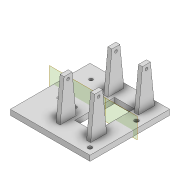
# Autodesk Inventor part: Motor_plate
Saved by Autodesk Inventor 2022 (Build 260153000, 153)
## iProperties
Created: 2022-08-27
Part Number: Motor_plate
Material: Generic
Document SubType Name: Modeling
Designer: dell
Density: 1 g/cm^3
Appearance: Default
Author: dell
Autodesk Inventor part; units mm, degrees
ref_plane "YZ Plane" through (0, 0, 0) normal (1, 0, 0) x (0, 1, 0)
ref_plane "XZ Plane" through (0, 0, 0) normal (0, 1, 0) x (-1, 0, 0)
ref_plane "XY Plane" through (0, 0, 0) normal (0, 0, 1) x (1, 0, 0)
sketch "Sketch1" plane through (0, 0, 0) normal (0, 1, 0) x (-1, 0, 0)
  line L0 (0, 0) -> (60, 0)
  line L1 (60, 0) -> (60, -60)
  line L2 (60, -60) -> (0, -60)
  line L3 (0, -60) -> (0, 0)
  circle A0 centre (37, -49.75) radius 1.3
  circle A1 centre (49, -49.75) radius 1.3
  circle A2 centre (37, -25.75) radius 1.3
  circle A3 centre (49, -25.75) radius 1.3
  circle A4 centre (5, -5) radius 1.55
  circle A5 centre (5, -40) radius 1.55
  dimension "d0" = 60
  dimension "d1" = 60
  dimension "d2" = 2.6
  dimension "d3" = 2.6
  dimension "d4" = 2.6
  dimension "d5" = 2.6
  dimension "d6" = 10.25
  dimension "d7" = 10.25
  dimension "d8" = 34.25
  dimension "d9" = 34.25
  dimension "d10" = 11
  dimension "d11" = 11
  dimension "d12" = 23
  dimension "d13" = 23
  dimension "d54" = 3.1
  dimension "d55" = 3.1
  dimension "d56" = 5
  dimension "d57" = 5
  dimension "d58" = 5
  dimension "d59" = 20
  constraints: 8 end point, 6 centre point, 2 parallel, 1 horizontal, 1 perpendicular
  measures "d0" distance of L2.end L0.start
  measures "d1" distance of L1.end L2.end
  measures "d2" diameter of A0
  measures "d3" diameter of A1
  measures "d4" diameter of A2
  measures "d5" diameter of A3
  measures "d6" distance from line of L2 A0.centre
  measures "d7" distance from line of L2 A1.centre
  measures "d8" distance from line of L2 A2.centre
  measures "d9" distance from line of L2 A3.centre
  measures "d10" distance from line of L1 A1.centre
  measures "d11" distance from line of L1 A3.centre
  measures "d12" distance from line of L1 A0.centre
  measures "d13" distance from line of L1 A2.centre
  measures "d54" diameter of A4
  measures "d55" diameter of A5
  measures "d56" distance from line of L0 A4.centre
  measures "d57" distance from line of L3 A4.centre
  measures "d58" distance from line of L3 A5.centre
  measures "d59" distance from line of L2 A5.centre
extrude "Extrusion1" add sketch "Sketch1" along normal blind 4
sketch "Sketch2" plane through (0, 4, 0) normal (0, 1, 0) x (1, 0, 0)
  line L0 (-13.5, 17) -> (-28.5, 17)
  line L1 (-28.5, 17) -> (-28.5, 47)
  line L2 (-28.5, 47) -> (-13.5, 47)
  line L3 (-13.5, 47) -> (-13.5, 17)
  line L4 (-13.5, 17) -> (-28.5, 47) construction
  line L5 (-28.5, 17) -> (-13.5, 47) construction
  line L6 (0, 60) -> (-60, 60) projected
  line L7 (-60, 60) -> (-60, 0) projected
  point P0 (0, 0)
  point P1 (-21, 32)
  dimension "d16" = 28
  dimension "d17" = 30
  dimension "d18" = 39
  dimension "d19" = 15
  constraints: 12 end point, 2 midpoint, 2 parallel, 1 horizontal, 1 perpendicular
  measures "d16" distance from line of L6 point (-21, 32)
  measures "d17" distance between parallel lines of L0 L2
  measures "d18" distance from line of L7 point (-21, 32)
  measures "d19" distance between parallel lines of L1 L3
extrude "Extrusion2" cut sketch "Sketch2" against normal blind 10
sketch "Sketch4" plane through (0, 4, 0) normal (0, 1, 0) x (1, 0, 0)
  line L0 (0, 60) -> (-60, 60) projected
  line L1 (-60, 60) -> (-60, 0) projected
  point P0 (0, 0)
  point P1 (-21, 32.5)
  dimension "d26" = 27.5
  dimension "d27" = 39
  measures "d26" distance from line of L0 point (-21, 32.5)
  measures "d27" distance from line of L1 point (-21, 32.5)
sketch "Sketch5" plane through (0, 4, 0) normal (0, 1, 0) x (1, 0, 0)
  line L0 (-34, 11.5) -> (-34, 17.5)
  line L1 (-34, 17.5) -> (-31, 17.5)
  line L2 (-31, 17.5) -> (-31, 11.5)
  line L3 (-31, 11.5) -> (-34, 11.5)
  line L4 (-11, 11.5) -> (-11, 17.5)
  line L5 (-11, 17.5) -> (-8, 17.5)
  line L6 (-8, 17.5) -> (-8, 11.5)
  line L7 (-8, 11.5) -> (-11, 11.5)
  point P0 (0, 0)
  point P1 (-21, 32.5)
  dimension "d28" = 3
  dimension "d29" = 3
  dimension "d30" = 15
  dimension "d31" = 6
  dimension "d32" = 10
  dimension "d33" = 10
  constraints: 16 end point, 4 parallel, 2 collinear, 2 perpendicular, 2 vertical
  measures "d28" distance of L0.end L1.end
  measures "d29" distance of L4.end L5.end
  measures "d30" distance from line of point (-21, 32.5) L1
  measures "d31" distance between parallel lines of L3 L1
  measures "d32" distance from line of point (-21, 32.5) L2
  measures "d33" distance from line of L4 point (-21, 32.5)
extrude "Extrusion4" add sketch "Sketch5" along normal blind 30
sketch "Sketch6" plane through (-8, 4, -11.5) normal (1, 0, 0) x (0, 0, -1)
  circle A0 centre (3, 27) radius 1.05
  line L0 (0, 0) -> (0, 30) projected
  line L1 (0, 30) -> (6, 30) projected
  point P0 (-11.5, -4)
  dimension "d36" = 2.1
  dimension "d37" = 3
  dimension "d38" = 3
  constraints: 1 centre point
  measures "d36" diameter of A0
  measures "d37" distance from line of L0 A0.centre
  measures "d38" distance from line of A0.centre L1
extrude "Extrusion5" cut sketch "Sketch6" against normal blind 100
chamfer "Chamfer1" distance 3 distance2 30 1 edges at (-32.5, 4, -11.5) measured on face at (-32.5, 4, -11)
chamfer "Chamfer2" distance 3 distance2 30 1 edges at (-9.5, 4, -11.5) measured on face at (-9.5, 4, -11)
chamfer "Chamfer3" distance 3 distance2 30 1 edges at (-32.5, 4, -17.5) measured on face at (-32.5, 4, -18)
chamfer "Chamfer4" distance 3 distance2 30 1 edges at (-9.5, 4, -17.5) measured on face at (-9.5, 4, -18)
ref_plane "Work Plane1" through (-21, 4, -32.5) normal (0, 0, -1) x (0, 1, 0)
mirror "Mirror1" about plane through (-21, 4, -32.5) normal (0, 0, -1) of "Extrusion5", "Extrusion4", "Chamfer3", "Chamfer1", "Chamfer2", "Chamfer4"
body "Solid1"
